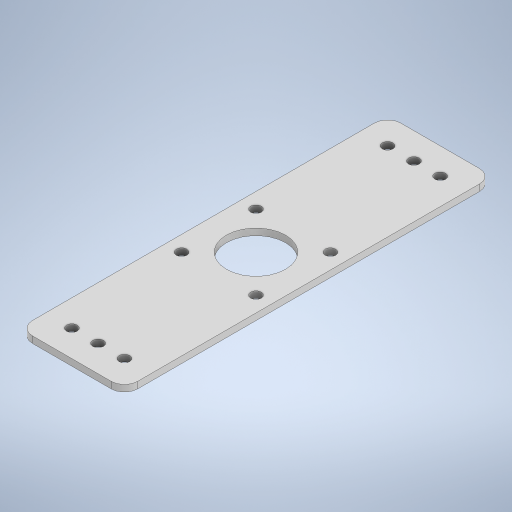
# Autodesk Inventor part: Shooter Sliding Motor Mount Plate V1.1
Saved by Autodesk Inventor 2024 (Build 280153000, 153)
## iProperties
Created: 2023-08-01
Part Number: Shooter Sliding Motor Mount Plate V1.1
Material: Generic
Document SubType Name: Modeling
Designer: Gabriel Marquez
Density: 1 g/cm^3
Appearance: Default
Author: Gabriel Marquez
Autodesk Inventor part; units mm, degrees
ref_plane "YZ Plane" through (0, 0, 0) normal (1, 0, 0) x (0, 1, 0)
ref_plane "XZ Plane" through (0, 0, 0) normal (0, 1, 0) x (-1, 0, 0)
ref_plane "XY Plane" through (0, 0, 0) normal (0, 0, 1) x (1, 0, 0)
sketch "Sketch1" plane through (0, 0, 0) normal (0, 1, 0) x (-1, 0, 0)
  circle A0 centre (0, 0) radius 25.4
  line L0 (17.9605, 17.9605) -> (-17.9605, 17.9605)
  line L1 (-17.9605, 17.9605) -> (-17.9605, -17.9605)
  line L2 (-17.9605, -17.9605) -> (17.9605, -17.9605)
  line L3 (17.9605, -17.9605) -> (17.9605, 17.9605)
  circle A1 centre (17.9605, 17.9605) radius 2.5797
  circle A2 centre (17.9605, -17.9605) radius 2.5797
  circle A3 centre (-17.9605, -17.9605) radius 2.5797
  circle A4 centre (-17.9605, 17.9605) radius 2.5797
  line L4 (-25.4, -63.5) -> (25.4, -63.5)
  line L5 (25.4, -63.5) -> (25.4, 63.5)
  line L6 (25.4, 63.5) -> (-25.4, 63.5)
  line L7 (-25.4, 63.5) -> (-25.4, -63.5)
  line L8 (25.4, 63.5) -> (-25.4, 63.5)
  line L9 (-25.4, 63.5) -> (-25.4, 88.9)
  line L10 (-25.4, 88.9) -> (25.4, 88.9)
  line L11 (25.4, 88.9) -> (25.4, 63.5)
  line L12 (25.4, -63.5) -> (-25.4, -63.5)
  line L13 (-25.4, -63.5) -> (-25.4, -88.9)
  line L14 (-25.4, -88.9) -> (25.4, -88.9)
  line L15 (25.4, -88.9) -> (25.4, -63.5)
  circle A5 centre (12.7, -76.2) radius 2.5797
  circle A6 centre (-12.7, -76.2) radius 2.5797
  circle A7 centre (0, -76.2) radius 2.5797
  circle A8 centre (-12.7, 76.2) radius 2.5797
  circle A9 centre (12.7, 76.2) radius 2.5797
  circle A10 centre (0, 76.2) radius 2.5797
  line L16 (-12.7, 76.2) -> (12.7, 76.2)
  line L17 (-12.7, -76.2) -> (12.7, -76.2)
  circle A11 centre (0, 0) radius 14.2875
  dimension "d0" = 50.8
  dimension "d1" = 5.1594
  dimension "d2" = 127
  dimension "d3" = 50.8
  dimension "d4" = 25.4
  dimension "d5" = 63.5
  dimension "d6" = 12.7
  dimension "d7" = 12.7
  dimension "d8" = 0
  dimension "d9" = 0
  dimension "d10" = 25.4
  dimension "d11" = 25.4
  dimension "d15" = 28.575
  constraints: 36 end point, 13 coincident, 12 centre point, 9 equal radius, 8 parallel, 6 horizontal, 4 equal length, 4 perpendicular, 3 point on circle, 2 midpoint
  measures "d0" diameter of A0
  measures "d1" diameter of A4
  measures "d2" distance of L6.end L4.start
  measures "d3" distance of L5.end L6.end
  measures "d4" distance from line of L7 point (0, 0)
  measures "d5" distance from line of point (0, 0) L6
  measures "d6" distance between parallel lines of L8 L16
  measures "d7" distance between parallel lines of L12 L17
  measures "d8" horizontal distance of point (0, 0) A10.centre
  measures "d9" horizontal distance of point (0, 0) point (0, -76.2)
  measures "d10" distance of L6.end L9.end
  measures "d11" distance of L16.start L16.end
  measures "d15" diameter of A11
extrude "Extrusion1" add sketch "Sketch1" along normal blind 3.175 contours A0 A2 L3 A1 | L5 L4 L7 A0 A3 A2 | A0 A1 A4 L7 L6 L5 | L15 L14 L13 L4 | L6 L9 L10 L11 | L3 A2 L2 A3 L1 A4 L0 A1 | A1 L0 A4 A0 | A0 A3 L2 A2 | A0 A4 L1 A3
fillet "Fillet1" radius 6.35 4 edges at (-25.4, 1.5875, 88.9) (25.4, 1.5875, 88.9) (25.4, 1.5875, -88.9) (-25.4, 1.5875, -88.9)
equation "\"d4\" = 0.5 * d3"
equation "\"d5\" = 0.5 * d2"
equation "\"d6\" = 0.5 * d10"
equation "\"d7\" = d6"
body "Solid1"
